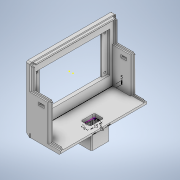
# Autodesk Inventor part: sUPORTE
Saved by Autodesk Inventor 2022 (Build 260153000, 153)
## iProperties
Created: 2022-12-13
Part Number: sUPORTE
Material: Genérico
Document SubType Name: Modeling
Designer: gugarauj07
Density: 1 g/cm^3
Appearance: Padrão
Author: gugarauj07
Autodesk Inventor part; units mm, degrees
ref_plane "YZ Plane" through (0, 0, 0) normal (1, 0, 0) x (0, 1, 0)
ref_plane "XZ Plane" through (0, 0, 0) normal (0, 1, 0) x (-1, 0, 0)
ref_plane "XY Plane" through (0, 0, 0) normal (0, 0, 1) x (1, 0, 0)
sketch "Esboço1" plane through (0, 0, 0) normal (1, 0, 0) x (0, 1, 0)
  line L0 (40.5, 60) -> (-42.5, 60)
  line L1 (-42.5, 60) -> (-42.5, -60)
  line L2 (-42.5, -60) -> (40.5, -60)
  line L3 (42.5, -58) -> (42.5, 58)
  line L4 (-42.5, 60) -> (42.5, -60) construction
  arc A0 (42.5, 58) -> (40.5, 60) centre (40.5, 58) ccw
  arc A1 (40.5, -60) -> (42.5, -58) centre (40.5, -58) ccw
  point P0 (0, 0)
  dimension "d0" = 85
  dimension "d1" = 120
  dimension "d4" = 2
  constraints: 10 end point, 4 point on circle, 4 tangent, 2 centre point, 2 parallel, 2 point on line, 1 equal radius, 1 horizontal, 1 midpoint, 1 perpendicular
  measures "d0" distance of L4.end L1.end
  measures "d1" distance of L0.end L1.end
  measures "d4" radius of A0
extrude "Extrusão1" add sketch "Esboço1" along normal blind 5
sketch "Esboço4" plane through (5, 0, 0) normal (1, 0, 0) x (0, 0, -1)
  line L0 (-60, -42.5) -> (60, -42.5) projected
  line L1 (-60, -42.5) -> (60, -42.5)
  line L2 (60, -42.5) -> (60, -47.5)
  line L3 (60, -47.5) -> (-60, -47.5)
  line L4 (-60, -47.5) -> (-60, -42.5)
  point P0 (0, 0)
  point P1 (60, -42.5)
  dimension "d33" = 5
  constraints: 8 end point, 2 parallel, 1 horizontal, 1 perpendicular
  measures "d33" distance of L1.end L2.end
extrude "Extrusão3" add sketch "Esboço4" against normal blind 5
sketch "Esboço5" plane through (5, 0, 0) normal (1, 0, 0) x (0, 0, -1)
  line L0 (-60, 40.5) -> (-60, -47.5) projected
  line L1 (60, 40.5) -> (60, -47.5) projected
  line L2 (-60, -47.5) -> (60, -47.5)
  line L3 (60, -47.5) -> (60, -42.5)
  line L4 (60, -42.5) -> (-60, -42.5)
  line L5 (-60, -42.5) -> (-60, -47.5)
  point P0 (0, 0)
  point P1 (60, -47.5)
  dimension "d36" = 5
  constraints: 8 end point, 2 parallel, 1 horizontal, 1 perpendicular, 1 point on line
  measures "d36" distance of L3.end L2.end
extrude "Extrusão4" add sketch "Esboço5" along normal blind 43
chamfer "Chanfro2" distance 4 angle 45 1 edges at (0, -47.5, 0)
chamfer "Chanfro3" distance 2 angle 45 1 edges at (48, -47.5, 0)
sketch "Esboço9" plane through (4, -47.5, -60) normal (0, -1, 0) x (1, 0, 0)
  line L0 (31, 50.5) -> (31, 47.5)
  line L1 (31, 69.5) -> (31, 72.5)
  line L2 (31, 72.5) -> (16.5, 72.5)
  line L3 (31, 47.5) -> (16.5, 47.5)
  line L4 (16.5, 47.5) -> (16.5, 72.5)
  line L5 (21.5, 67.5) -> (21.5, 52.5) projected
  arc A0 (21.5, 52.5) -> (23.5, 50.5) centre (23.5, 52.5) ccw projected
  arc A1 (21.5, 52.5) -> (23.5, 50.5) centre (23.5, 52.5) ccw
  arc A2 (23.5, 69.5) -> (21.5, 67.5) centre (23.5, 67.5) ccw
  arc A3 (34.5, 67.5) -> (32.5, 69.5) centre (32.5, 67.5) ccw
  line L6 (23.5, 69.5) -> (32.5, 69.5)
  line L7 (23.5, 50.5) -> (32.5, 50.5)
  line L8 (34.5, 67.5) -> (34.5, 52.5)
  arc A4 (32.5, 50.5) -> (34.5, 52.5) centre (32.5, 52.5) ccw
  line L9 (34.5, 55.3451) -> (39.5, 55.3451)
  line L10 (31, 47.5) -> (39.5, 47.5)
  line L11 (39.5, 47.5) -> (39.5, 72.5)
  line L12 (39.5, 72.5) -> (31, 72.5)
  point P0 (-4, 60)
  point P1 (32.5, 50.5)
  dimension "d230" = 15
  dimension "d231" = 9
  dimension "d232" = 9
  dimension "d233" = 15
  dimension "d235" = 5
  dimension "d236" = 25
  constraints: 24 end point, 8 point on circle, 5 perpendicular, 4 centre point, 3 horizontal, 3 point on line, 3 vertical, 2 tangent
  measures "d230" distance of L5.start L5.end
  measures "d231" distance of L6.start L6.end
  measures "d232" distance of L7.start point (32.5, 50.5)
  measures "d233" distance of L8.start point (34.5, 52.5)
  measures "d235" distance of L9.start L9.end
  measures "d236" distance of L10.end L11.end
extrude "Extrusão7" add sketch "Esboço9" along normal blind 21 contours L7 A4 L8 L9 L11 L10 L0 | L0 L3 L4 L2 L1 L6 A2 L5 A0 L7 | L9 L8 A3 L6 L1 L12 L11
fillet "Arredondamento1" radius 2 4 edges at (20.5, -58, -12.5) (20.5, -58, 12.5) (43.5, -58, -12.5) (43.5, -58, 12.5)
sketch "Esboço12" plane through (5, 0, 0) normal (1, 0, 0) x (0, 0, -1)
  line L0 (60, -42.5) -> (60, 40.5) projected
  line L1 (60, -42.5) -> (55, -42.5)
  line L2 (55, -42.5) -> (55, 7.5)
  line L3 (55, 7.5) -> (60, 7.5)
  line L4 (60, 7.5) -> (60, -42.5)
  line L5 (60, -42.5) -> (-60, -42.5) projected
  line L6 (-60, -42.5) -> (-55, -42.5)
  line L7 (-55, -42.5) -> (-55, 7.5)
  line L8 (-55, 7.5) -> (-60, 7.5)
  line L9 (-60, 7.5) -> (-60, -42.5)
  point P0 (0, 0)
  dimension "d123" = 5
  dimension "d124" = 50
  dimension "d125" = 5
  dimension "d126" = 50
  constraints: 16 end point, 4 parallel, 2 horizontal, 2 perpendicular
  measures "d123" distance of L2.end L3.end
  measures "d124" distance of L1.end L2.end
  measures "d125" distance of L8.end L7.end
  measures "d126" distance of L7.end L6.end
extrude "Extrusão10" add sketch "Esboço12" along normal blind 25
sketch "Esboço13" plane through (30, 0, 0) normal (1, 0, 0) x (0, 0, -1)
  line L0 (-60, 40.5) -> (-60, -43.5) projected
  line L1 (-60, -42.5141) -> (-58.4, -42.5141)
  line L2 (-60, -42.5141) -> (-58.4, -42.5141) construction
  line L3 (-55, 7.5) -> (-60, 7.5) projected
  line L4 (58, 42.5) -> (-58, 42.5) projected
  line L5 (-57.5, 42.5) -> (-56, 42.5) construction
  line L6 (60, -42.5) -> (55, -42.5) projected
  line L7 (60, -42.5) -> (58.4, -42.5)
  line L8 (55, 7.5) -> (60, 7.5) projected
  line L9 (-55, -42.5) -> (-60, -42.5) projected
  line L10 (-58.4, -42.5) -> (-56.6, -42.5)
  line L11 (-56.6, -42.5) -> (-56.6, 7.5)
  line L12 (-56.6, 7.5) -> (-58.4, 7.5)
  line L13 (-58.4, 7.5) -> (-58.4, -42.5)
  line L14 (60, 7.5) -> (55, 7.5) projected
  line L15 (58.4, -42.5) -> (56.6, -42.5)
  line L16 (56.6, -42.5) -> (56.6, 7.5)
  line L17 (56.6, 7.5) -> (58.4, 7.5)
  line L18 (58.4, 7.5) -> (58.4, -42.5)
  point P0 (0, 0)
  dimension "d129" = 1.6
  dimension "d130" = 0
  dimension "d135" = 1.6
  dimension "d240" = 1.8
  dimension "d241" = 1.8
  constraints: 24 end point, 6 point on line, 4 horizontal, 4 parallel, 3 perpendicular, 1 collinear
  measures "d129" distance of L1.start L1.end
  measures "d130" distance between parallel lines of L1 L2
  measures "d135" distance of L6.start L7.end
  measures "d240" distance of L12.end L11.end
  measures "d241" distance of L16.end L17.end
extrude "Extrusão11" add sketch "Esboço13" along normal blind 4 contours L3 L11 L9 L13 | L6 L16 L8 L18
extrude "Extrusão12" cut sketch "Esboço9" along normal blind 21 contours L7 A0 L5 A2 L6 A3 L8 A4
sketch "Esboço14" plane through (5, 0, 0) normal (1, 0, 0) x (0, 0, -1)
  line L0 (-55, 7.5) -> (-60, 7.5) projected
  line L1 (-58.5, 7.5) -> (-56.5, 7.5)
  line L2 (58.5055, 7.5) -> (56.5055, 7.5)
  line L3 (56.5055, 41) -> (56.5055, 41)
  line L4 (60, 7.5) -> (58.4, 7.5)
  line L5 (55, -42.5) -> (55, 7.5) projected
  line L6 (55, 7.5) -> (56.6, 7.5)
  line L7 (55, 7.5) -> (60, 7.5) projected
  line L8 (58.4, 7.5) -> (56.6, 7.5)
  line L9 (56.6, 7.5) -> (56.6, 40.9978)
  line L10 (58.4, 40.9978) -> (58.4, 7.5)
  line L11 (-60, 7.5) -> (-58.4, 7.5)
  line L12 (-54.9942, 7.5) -> (-56.5942, 7.5)
  line L13 (-56.6, 7.5) -> (-58.4, 7.5) projected
  line L14 (58, 42.5) -> (-58, 42.5) projected
  line L15 (-56.5942, 7.5) -> (-58.3942, 7.5)
  line L16 (-58.3942, 7.5) -> (-58.3942, 40.9)
  line L17 (-58.3942, 40.9) -> (-56.5942, 40.9)
  line L18 (-56.5942, 40.9) -> (-56.5942, 7.5)
  line L19 (-60, 40.5) -> (-60, 7.5) projected
  line L20 (-56.3942, 40.9) -> (56.4, 40.9)
  line L21 (58.4, 38.9) -> (58.4, 39.1)
  line L22 (58.4, 39.1) -> (-58.3942, 39.1)
  line L23 (-58.3942, 39.1) -> (-58.3942, 38.9)
  arc A0 (-56.3942, 40.9) -> (-58.3942, 38.9) centre (-56.3942, 38.9) ccw
  arc A1 (58.4, 38.9) -> (56.4, 40.9) centre (56.4, 38.9) ccw
  point P0 (0, 0)
  point P1 (58.4, 40.9)
  point P2 (-56.5942, 39.1)
  point P3 (56.6, 39.1)
  point P4 (-56.5942, 40.89)
  dimension "d214" = 1.6
  dimension "d215" = 1.6
  dimension "d216" = 1.8
  dimension "d218" = 1.6
  dimension "d221" = 1.6058
  dimension "d222" = 1.8
  dimension "d223" = 2
  dimension "d224" = 2
  constraints: 36 end point, 8 point on line, 6 parallel, 5 horizontal, 4 point on circle, 4 tangent, 3 perpendicular, 2 centre point
  measures "d214" distance of L4.start L4.end
  measures "d215" distance of L5.end L6.end
  measures "d216" distance between parallel lines of L9 L10
  measures "d218" distance of L12.start L12.end
  measures "d221" distance between parallel lines of L19 L16
  measures "d222" distance of point (58.4, 40.9) L21.end
  measures "d223" radius of A0
  measures "d224" radius of A1
extrude "Extrusão13" add sketch "Esboço14" along normal blind 4 contours L0 L16 A0 L22 L18 | L22 A0 L18 | L18 A0 L20 A1 L9 L22 | A0 L22 L16 L17 L18 | L22 A1 L10 L2 L9 | L9 A1 L22 | A0 L16 L22
sketch "Esboço15" plane through (9, 0, 0) normal (1, 0, 0) x (0, 0, -1)
  line L0 (-56.5942, 7.5) -> (-58.3942, 7.5) projected
  line L1 (-56.5942, 7.5) -> (-56.5942, 39.1) projected
  line L2 (-58.3942, 7.5) -> (-56.5942, 7.5)
  line L3 (-56.5942, 7.5) -> (-56.5942, 10.5)
  line L4 (-56.5942, 10.5) -> (-58.3942, 10.5)
  line L5 (-58.3942, 10.5) -> (-58.3942, 7.5)
  line L6 (58.4, 38.9) -> (58.4, 7.5) projected
  line L7 (56.6, 7.5) -> (56.6, 39.1) projected
  line L8 (58.4, 7.5) -> (56.6, 7.5)
  line L9 (56.6, 7.5) -> (56.6, 10.5)
  line L10 (56.6, 10.5) -> (58.4, 10.5)
  line L11 (58.4, 10.5) -> (58.4, 7.5)
  point P0 (0, 0)
  point P1 (-56.5, 7.5)
  point P2 (58.5, 7.5)
  point P3 (56.5, 7.5)
  dimension "d239" = 3
  dimension "d242" = 3
  constraints: 16 end point, 4 parallel, 2 horizontal, 2 perpendicular, 2 point on line
  measures "d239" distance of L3.end L2.end
  measures "d242" distance of L8.end L9.end
extrude "Extrusão14" add sketch "Esboço15" along normal blind 25
sketch "Esboço16" plane through (34, 0, 0) normal (1, 0, 0) x (0, 0, -1)
  line L0 (-56.6, -42.5) -> (-58.4, -42.5) projected
  line L1 (-56.5, -42.5) -> (-58.5, -42.5)
  line L2 (60, -42.5) -> (55, -42.5) projected
  line L3 (58.5, -42.5) -> (56.5, -42.5)
  line L4 (-56.6, 7.5) -> (-56.6, -42.5) projected
  line L5 (-58.4, 7.5) -> (-58.4, -42.5) projected
  line L6 (-56.6, -42.5) -> (-58.4, -42.5)
  line L7 (-58.4, -42.5) -> (-58.4, -39.5)
  line L8 (-58.4, -39.5) -> (-56.6, -39.5)
  line L9 (-56.6, -39.5) -> (-56.6, -42.5)
  line L10 (58.4, -42.5) -> (56.6, -42.5) projected
  line L11 (56.6, 10.5) -> (56.6, -42.5) projected
  line L12 (58.4, -42.5) -> (56.6, -42.5)
  line L13 (56.6, -42.5) -> (56.6, -39.5)
  line L14 (56.6, -39.5) -> (58.4, -39.5)
  line L15 (58.4, -39.5) -> (58.4, -42.5)
  point P0 (0, 0)
  dimension "d243" = 3
  dimension "d244" = 3
  constraints: 20 end point, 4 horizontal, 4 parallel, 2 perpendicular, 2 point on line
  measures "d243" distance of L6.end L7.end
  measures "d244" distance of L12.end L13.end
extrude "Extrusão15" add sketch "Esboço16" along normal blind 14
chamfer "Chanfro4" distance 2 angle 45 2 edges at (48, -39.5, 57.5) (48, -39.5, -57.5)
chamfer "Chanfro5" distance 2 angle 45 2 edges at (34, 10.5, -57.5) (34, 10.5, 57.4942)
sketch "Esboço17" plane through (9, 0, 0) normal (1, 0, 0) x (0, 0, -1)
  line L0 (-60, 42.5) -> (-57, 42.5)
  line L1 (-57, 42.5) -> (-57, 39.5)
  line L2 (-57, 39.5) -> (-60, 39.5)
  line L3 (-60, 39.5) -> (-60, 42.5)
  line L4 (60, 42.5) -> (57, 42.5)
  line L5 (57, 42.5) -> (57, 39.5)
  line L6 (57, 39.5) -> (60, 39.5)
  line L7 (60, 39.5) -> (60, 42.5)
  point P0 (0, 0)
  dimension "d166" = 3
  dimension "d167" = 3
  dimension "d168" = 3
  dimension "d169" = 3
  constraints: 16 end point, 4 parallel, 2 horizontal, 2 perpendicular
  measures "d166" distance of L1.end L2.end
  measures "d167" distance of L0.end L1.end
  measures "d168" distance of L6.end L5.end
  measures "d169" distance of L5.end L4.end
hole "Furo5" at (9, 39.5, 57) at (9, 39.5, -57) direction (-1, 0, 0) diameter 4.3434 depth 16.265 tip angle 118 thread size "12-24 UNC" class "2B" standard "ANSI Unified Screw Threads"
sketch "Esboço18" plane through (4, -68.5, -60) normal (0, -1, 0) x (1, 0, 0)
  line L0 (21.5, 102.5) -> (21.5, 87.5) projected
  line L1 (21.5, 102.5) -> (21.5, 101.5)
  line L2 (21.5, 101.5) -> (19.5, 101.5)
  line L3 (19.5, 101.5) -> (19.5, 88.5)
  line L4 (19.5, 88.5) -> (21.5, 88.5)
  line L5 (21.5, 88.5) -> (21.5, 101.5)
  arc A0 (23.5, 69.5) -> (21.5, 67.5) centre (23.5, 67.5) ccw projected
  line L6 (21.5, 67.5) -> (21.5, 66.5)
  line L7 (21.5, 67.5) -> (21.5, 52.5) projected
  line L8 (21.5, 66.5) -> (19.5, 66.5)
  line L9 (19.5, 66.5) -> (19.5, 53.5)
  line L10 (19.5, 53.5) -> (21.5, 53.5)
  line L11 (21.5, 53.5) -> (21.5, 66.5)
  line L12 (21.5, 32.5) -> (21.5, 17.5) projected
  line L13 (21.5, 32.5) -> (21.5, 31.5)
  line L14 (21.5, 31.5) -> (19.5, 31.5)
  line L15 (19.5, 31.5) -> (19.5, 18.5)
  line L16 (19.5, 18.5) -> (21.5, 18.5)
  line L17 (21.5, 18.5) -> (21.5, 31.5)
  point P0 (-4, 60)
  point P1 (21.5, 18.5)
  dimension "d177" = 1
  dimension "d178" = 2
  dimension "d179" = 13
  dimension "d180" = 1
  dimension "d181" = 2
  dimension "d182" = 13
  dimension "d183" = 1
  dimension "d184" = 13
  constraints: 30 end point, 6 parallel, 3 horizontal, 3 perpendicular, 3 point on line
  measures "d177" distance of L0.start L1.end
  measures "d178" distance of L4.end L3.end
  measures "d179" distance of L3.end L2.end
  measures "d180" distance of L6.start L6.end
  measures "d181" distance of L10.end L9.end
  measures "d182" distance of L9.end L8.end
  measures "d183" distance of L12.start L13.end
  measures "d184" distance of L15.end L14.end
extrude "Extrusão16" cut sketch "Esboço18" against normal blind 19
sketch "Esboço21" plane through (0, 40.5, 60) normal (0, 0, 1) x (1, 0, 0)
  line L0 (17, -43) -> (25, -43)
  line L1 (25, -43) -> (25, -39)
  line L2 (25, -39) -> (17, -39)
  line L3 (17, -39) -> (17, -43)
  point P0 (0, -40.5)
  point P1 (30, -33)
  dimension "d195" = 8
  dimension "d196" = 4
  constraints: 8 end point, 2 parallel, 1 horizontal, 1 perpendicular
  measures "d195" distance of L2.end L1.end
  measures "d196" distance of L1.end L0.end
extrude "Extrusão18" cut sketch "Esboço21" against normal through all
sketch "Esboço22" plane through (5, 0, 0) normal (1, 0, 0) x (0, 0, -1)
  line L0 (43.5, -28) -> (-43.5, -28)
  line L1 (-43.5, -28) -> (-43.5, 28)
  line L2 (-43.5, 28) -> (43.5, 28)
  line L3 (43.5, 28) -> (43.5, -28)
  line L4 (43.5, -28) -> (-43.5, 28) construction
  line L5 (-43.5, -28) -> (43.5, 28) construction
  point P0 (0, 0)
  dimension "d199" = 87
  dimension "d200" = 56
  constraints: 12 end point, 2 midpoint, 2 parallel, 1 horizontal, 1 perpendicular
  measures "d199" distance of L1.end L2.end
  measures "d200" distance of L0.end L1.end
extrude "Extrusão19" cut sketch "Esboço22" against normal through all
sketch "Esboço23" plane through (5, 0, 0) normal (1, 0, 0) x (0, 0, -1)
  line L0 (-43.5, -28) -> (-43.5, 28) projected
  line L1 (-43.5, 28) -> (-51.5, 28)
  line L2 (-51.5, 28) -> (-51.5, -28)
  line L3 (-51.5, -28) -> (-43.5, -28)
  line L4 (-43.5, -28) -> (-43.5, 28)
  line L5 (43.5, 28) -> (43.5, -28) projected
  line L6 (43.5, -28) -> (51.5, -28)
  line L7 (51.5, -28) -> (51.5, 28)
  line L8 (51.5, 28) -> (43.5, 28)
  line L9 (43.5, 28) -> (43.5, -28)
  point P0 (0, 0)
  dimension "d203" = 8
  dimension "d204" = 8
  constraints: 16 end point, 4 parallel, 2 horizontal, 2 perpendicular, 1 point on line
  measures "d203" distance of L3.end L2.end
  measures "d204" distance of L8.end L7.end
extrude "Extrusão20" cut sketch "Esboço23" against normal blind 3
sketch "Esboço24" plane through (2, 0, 0) normal (1, 0, 0) x (0, 0, -1)
  line L0 (51.5, -28) -> (-51.5, -28) projected
  line L1 (-51.5, -28) -> (-47.5, -28)
  circle A0 centre (-47.5, -24) radius 1.5
  line L2 (-43.5, -28) -> (43.5, -28) projected
  line L3 (43.5, 28) -> (-43.5, 28) projected
  circle A1 centre (47.5, -24) radius 1.5
  line L4 (-51.5, -28) -> (-51.5, 28) projected
  line L5 (51.5, 28) -> (51.5, -28) projected
  circle A2 centre (-47.5, 24) radius 1.5
  circle A3 centre (47.5, 24) radius 1.5
  dimension "d209" = 3
  constraints: 4 centre point, 2 end point, 1 horizontal
  measures "d209" diameter of A0
extrude "Extrusão21" cut sketch "Esboço24" against normal through all
extrude "Extrusão23" cut sketch "Esboço9" against normal through all contours L7 A0 L5 A2 L6 A3 L8 A4
fillet "Arredondamento2" radius 0.8 27 edges at (47, -40.5, 56.6) (47, -40.5, 58.4) (40, -39.5, 56.6) (40, -39.5, 58.4) (34, -16, 56.6) (34, -16, 58.4) (34, 8, 56.5942) (33, 9.5, 56.5942) (33, 9.5, 58.3942) (20.5, 10.5, 56.5942) (20.5, 10.5, 58.3942) (9, 23.9333, 56.5942) (9, 24.1675, 58.3942) (9, 39.1, 0) (9, 40.9, 0) (40, -39.5, -58.4) (40, -39.5, -56.6) (47, -40.5, -58.4) (47, -40.5, -56.6) (34, -15.5, -58.4) (34, -15.5, -56.6) (20.5, 10.5, -58.4) (20.5, 10.5, -56.6) (33, 9.5, -58.4) (33, 9.5, -56.6) (9, 24.1699, -58.4) (9, 23.9327, -56.6)
sketch "Esboço25" plane through (0, 0, 0) normal (-1, 0, 0) x (0, 0, 1)
  point P0 (0, 0)
